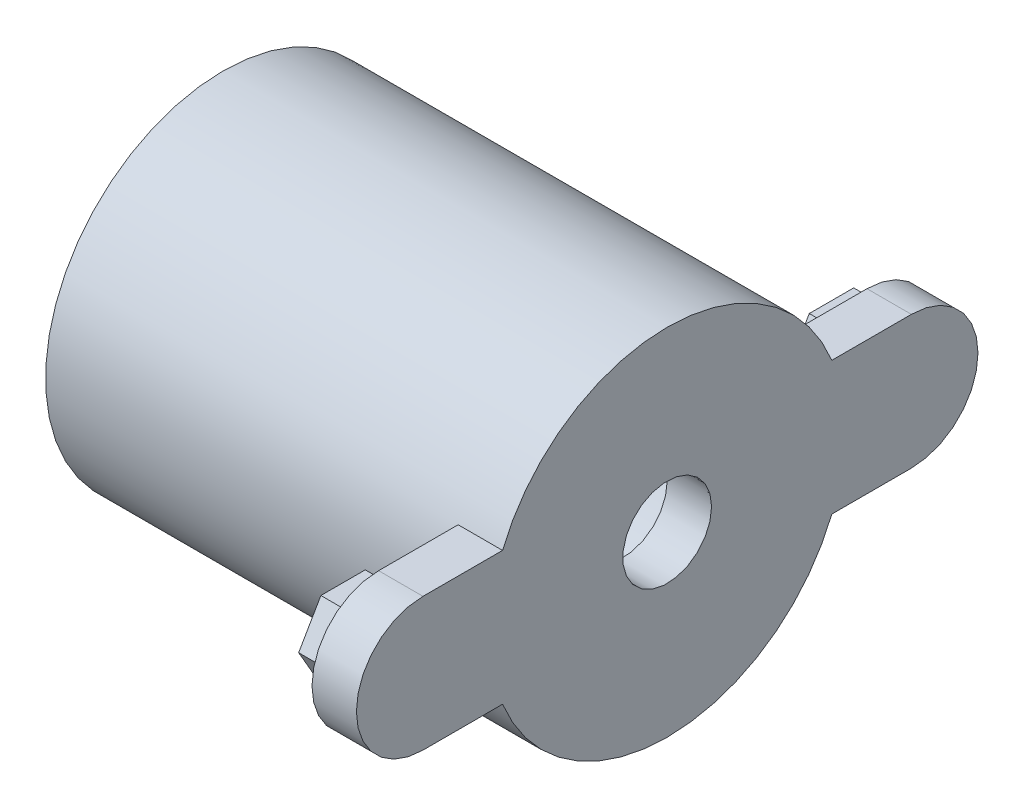
# Autodesk Inventor part: Cylinder
Saved by Autodesk Inventor 2021 (Build 250183000, 183)
## iProperties
Created: 2015-03-05
Part Number: Cylinder
Document SubType Name: Modeling
Designer: Administrator
Density: 1 g/cm^3
Mass: 0.29412 g
Surface Area: 6.12533 cm^2
Volume: 0.29412 cm^3
Material: Generic
Appearance: Cool White
Author: Administrator
Autodesk Inventor part; units mm, degrees
ref_plane "YZ Plane" through (0, 0, 0) normal (1, 0, 0) x (0, 1, 0)
ref_plane "XZ Plane" through (0, 0, 0) normal (0, 1, 0) x (-1, 0, 0)
ref_plane "XY Plane" through (0, 0, 0) normal (0, 0, 1) x (1, 0, 0)
sketch "Sketch1" plane through (0, 0, 0) normal (0, 0, 1) x (1, 0, 0)
  line L0 (0, 0) -> (0, 4) construction
  line L1 (0, 4) -> (5, 4)
  line L2 (5, 4) -> (5, 0)
  line L3 (5, 0) -> (4, 0)
  line L4 (4, 0) -> (4, 3)
  line L5 (4, 3) -> (0, 3)
  line L6 (0, 0) -> (55.2609, 0) construction
  line L7 (0, 4) -> (-5, 4)
  line L8 (-5, 4) -> (-5, 0) construction
  line L9 (-4, 0) -> (-4, 3) construction
  line L10 (-4, 3) -> (0, 3)
  line L11 (-5, 1.5) -> (-4, 1.5)
  line L12 (-5, 1.5) -> (-5, 4)
  line L13 (-4, 1.5) -> (-4, 3)
  dimension "d0" = 1
  dimension "d1" = 3
  dimension "d2" = 0
  dimension "d3" = 1
  dimension "d4" = 5
  dimension "d5" = 1.5
  constraints: 28 end point, 5 parallel, 4 symmetric about line, 2 collinear, 2 perpendicular, 2 point on line, 1 midpoint, 1 vertical, 1 other
  measures "d0" distance between parallel lines of L1 L5
  measures "d1" distance between parallel lines of L5 L3
  measures "d2" distance between parallel lines of L3 L6
  measures "d3" distance between parallel lines of L4 L2
  measures "d4" distance between parallel lines of L0 L2
  measures "d5" distance between parallel lines of L11 L6
revolve "Revolution1" add sketch "Sketch1" angle 360 about axis through (0, 0, 0) along (1, 0, 0)
sketch "Sketch6" plane through (5, 0, 0) normal (1, 0, 0) x (0, 0, -1)
  line L0 (0, 0) -> (-7, 0) construction
  line L1 (-7, 0) -> (-7, 1.5)
  line L2 (-7, 1.5) -> (-3.4641, 1.5)
  line L3 (0, 0) -> (0, 4) construction
  line L4 (-7, 0) -> (-7, -1.5)
  line L5 (-7, -1.5) -> (-3.4641, -1.5)
  line L6 (0, 0) -> (7, 0) construction
  line L7 (7, 0) -> (7, 1.5)
  line L8 (7, 1.5) -> (3.4641, 1.5)
  line L9 (7, 0) -> (7, -1.5)
  line L10 (7, -1.5) -> (3.4641, -1.5)
  arc A0 (-3.4641, 1.5) -> (-3.4641, -1.5) centre (0, 0) ccw construction
  arc A1 (3.4641, -1.5) -> (3.4641, 1.5) centre (0, 0) ccw construction
  line L11 (-7, -1.5) -> (-7, 1.5) construction
  line L12 (7, -1.5) -> (7, 1.5) construction
  line L13 (-7, 1.5) -> (7, 1.5)
  line L14 (-7, -1.5) -> (7, -1.5)
  dimension "d30" = 1.5
  dimension "d31" = 7
  constraints: 30 end point, 7 symmetric about line, 4 collinear, 4 point on circle, 2 centre point, 2 perpendicular, 1 coincident, 1 horizontal, 1 parallel
  measures "d30" distance between parallel lines of L2 L0
  measures "d31" distance between parallel lines of L1 L3
extrude "Extrusion5" add sketch "Sketch6" against normal blind 1
fillet "Fillet2" radius 1.5 4 edges at (4.5, -1.5, 7) (4.5, 1.5, 7) (4.5, -1.5, -7) (4.5, 1.5, -7)
sketch "Sketch7" plane through (4, 0, 0) normal (-1, 0, 0) x (0, 0, 1)
  arc A0 (5.5, -1.5) -> (5.5, 1.5) centre (5.5, 0) ccw projected
  arc A1 (-5.5, 1.5) -> (-5.5, -1.5) centre (-5.5, 0) ccw projected
  line L0 (-3.7081, -1.5) -> (-5.5, -1.5) projected
  arc A2 (-3.7081, 1.5) -> (-3.7081, -1.5) centre (0, 0) ccw projected
  line L1 (-5.5, 1.5) -> (-3.7081, 1.5) projected
  line L2 (6, 0.866) -> (6.5, 0)
  line L3 (6.5, 0) -> (6, -0.866)
  line L4 (6, -0.866) -> (5, -0.866)
  line L5 (5, -0.866) -> (4.5, 0)
  line L6 (4.5, 0) -> (5, 0.866)
  line L7 (5, 0.866) -> (6, 0.866)
  line L8 (-5, 0.866) -> (-4.5, 0)
  line L9 (-4.5, 0) -> (-5, -0.866)
  line L10 (-5, -0.866) -> (-6, -0.866)
  line L11 (-6, -0.866) -> (-6.5, 0)
  line L12 (-6.5, 0) -> (-6, 0.866)
  line L13 (-6, 0.866) -> (-5, 0.866)
  dimension "d35" = 1
  constraints: 24 end point, 2 coincident, 1 collinear, 26 other
  measures "d35" distance of L12.end L8.start
extrude "Extrusion6" add sketch "Sketch7" along normal blind 0.8 contours L2 L3 L4 L5 L6 L7 | L8 L9 L10 L11 L12 L13
sketch "Sketch8" plane through (5, 0, 0) normal (1, 0, 0) x (0, 0, -1)
  arc A0 (3.7081, 1.5) -> (-3.7081, 1.5) centre (0, 0) ccw projected
  circle A1 centre (0, 0) radius 1
  dimension "d38" = 2
  constraints: 1 centre point, 1 coincident
  measures "d38" diameter of A1
extrude "Extrusion7" cut sketch "Sketch8" against normal blind 10
sketch "Sketch9" plane through (-5, 0, 0) normal (-1, 0, 0) x (0, 0, 1)
  circle A0 centre (0, 0) radius 1.5 projected
extrude "Extrusion8" add sketch "Sketch9" against normal blind 1
body "Solid1"
